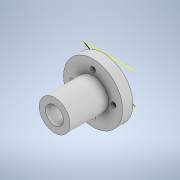
# Autodesk Inventor part: axis
Saved by Autodesk Inventor 2022 (Build 260153000, 153)
## iProperties
Created: 2023-10-26
Part Number: axis
Material: Generisch
Document SubType Name: Modeling
Designer: Marc Panse
Density: 1 g/cm^3
Appearance: Vorgabe
Author: Marc Panse
## iProperties of the stored document LCDmount_3D-Druck.ipt
Created: 2023-10-26
Part Number: LCDmount_3D-Druck
Material: Generisch
Document SubType Name: Modeling
Designer: Marc Panse
Density: 1 g/cm^3
Appearance: Vorgabe
Author: Marc Panse
Autodesk Inventor part; units mm, degrees
ref_plane "YZ Plane" through (0, 0, 0) normal (1, 0, 0) x (0, 1, 0)
ref_plane "XZ Plane" through (0, 0, 0) normal (0, 1, 0) x (-1, 0, 0)
ref_plane "XY Plane" through (0, 0, 0) normal (0, 0, 1) x (1, 0, 0)
sketch "Skizze1" plane through (0, 0, 0) normal (0, 0, 1) x (1, 0, 0)
  circle A0 centre (0, 0) radius 18
  circle A1 centre (0, 0) radius 25
  dimension "d0" = 36
  dimension "d1" = 50
  constraints: 2 centre point, 2 coincident
  measures "d0" diameter of A0
  measures "d1" diameter of A1
extrude "Extrusion1" add sketch "Skizze1" along normal blind 35
sketch "Skizze2" plane through (0, 0, 35) normal (0, 0, 1) x (1, 0, 0)
  circle A0 centre (0, 0) radius 19.3
  line L0 (0, -19.3) -> (0, -21.4)
  line L1 (0, -21.4) -> (-7.65, -21.4)
  line L2 (-7.65, -21.4) -> (7.65, -21.4)
  line L3 (7.65, -21.4) -> (7.65, -17.7191)
  line L4 (-7.65, -21.4) -> (-7.65, -17.7191)
  circle A1 centre (0, 0) radius 25 projected
  circle A2 centre (0, 0) radius 18 projected
  circle A3 centre (0, 0) radius 25 projected
  circle A4 centre (0, 0) radius 18 projected
  circle A5 centre (0, 0) radius 19.3
  dimension "d4" = 38.6
  dimension "d5" = 2.1
  dimension "d6" = 7.65
  dimension "d7" = 90
  dimension "d8" = 15.3
  constraints: 10 end point, 3 point on circle, 2 centre point, 2 coincident, 2 perpendicular, 1 concentric, 1 parallel, 1 point on line, 1 vertical
  measures "d4" diameter of A0
  measures "d5" distance of L0.start L0.end
  measures "d6" distance of L0.end L1.end
  measures "d7" angle of L0 L1
  measures "d8" distance of L1.end L2.end
extrude "Extrusion2" cut sketch "Skizze2" against normal blind 34 contours A0 | A0 L0 L1 L4 | L3 L2 L0 A0 | A2
fillet "Rundung1" radius 4 2 edges at (-7.65, -17.7191, 18) (7.65, -17.7191, 18)
sketch "Skizze3" plane through (0, 0, 35) normal (0, 0, 1) x (1, 0, 0)
  arc A0 (9.65, -16.7143) -> (7.65, -20.1784) centre (11.65, -20.1784) ccw projected
  line L0 (7.65, -20.1784) -> (7.65, -21.4) projected
  line L1 (7.65, -21.4) -> (-7.65, -21.4) projected
  line L2 (-7.65, -21.4) -> (-7.65, -20.1784) projected
  arc A1 (-7.65, -20.1784) -> (-9.65, -16.7143) centre (-11.65, -20.1784) ccw projected
  arc A2 (9.65, -16.7143) -> (-9.65, -16.7143) centre (0, 0) ccw projected
  circle A3 centre (0, 0) radius 25 projected
extrude "Extrusion3" cut sketch "Skizze3" against normal blind 25
sketch "Skizze4" plane through (0, 0, 10) normal (0, 0, 1) x (1, 0, 0)
  circle A0 centre (0, 0) radius 24
  circle A1 centre (0, 0) radius 25 projected
  arc A2 (9.65, -16.7143) -> (7.65, -20.1784) centre (11.65, -20.1784) ccw projected
  line L0 (7.65, -21.4) -> (7.65, -20.1784) projected
  line L1 (-7.65, -21.4) -> (7.65, -21.4) projected
  line L2 (-7.65, -20.1784) -> (-7.65, -21.4) projected
  arc A3 (-7.65, -20.1784) -> (-9.65, -16.7143) centre (-11.65, -20.1784) ccw projected
  arc A4 (9.65, -16.7143) -> (-9.65, -16.7143) centre (0, 0) ccw projected
  dimension "d14" = 48
  constraints: 1 centre point, 1 coincident
  measures "d14" diameter of A0
extrude "Extrusion4" cut sketch "Skizze4" against normal blind 9.25 contours A1
sketch "Skizze5" plane through (0, 0, 10) normal (0, 0, 1) x (1, 0, 0)
  circle A0 centre (0, 0) radius 24 projected
  arc A1 (9.65, -16.7143) -> (7.65, -20.1784) centre (11.65, -20.1784) ccw projected
  line L0 (7.65, -21.4) -> (7.65, -20.1784) projected
  line L1 (-7.65, -21.4) -> (7.65, -21.4) projected
  line L2 (-7.65, -20.1784) -> (-7.65, -21.4) projected
  arc A2 (-7.65, -20.1784) -> (-9.65, -16.7143) centre (-11.65, -20.1784) ccw projected
  arc A3 (9.65, -16.7143) -> (-9.65, -16.7143) centre (0, 0) ccw projected
extrude "Extrusion5" cut sketch "Skizze5" against normal blind 2.2
sketch "Skizze6" plane through (0, 0, 7.8) normal (0, 0, 1) x (1, 0, 0)
  line L0 (30, -2.706) -> (-30, -2.706)
  line L1 (-30, -2.706) -> (-30, 2.706)
  line L2 (-30, 2.706) -> (30, 2.706)
  line L3 (30, 2.706) -> (30, -2.706)
  line L4 (30, -2.706) -> (-30, 2.706) construction
  line L5 (-30, -2.706) -> (30, 2.706) construction
  point P0 (0, 0)
  dimension "d33" = 60
  constraints: 12 end point, 2 midpoint, 2 parallel, 1 horizontal, 1 perpendicular
  measures "d33" distance between parallel lines of L3 L1
extrude "Extrusion6" cut sketch "Skizze6" against normal blind 2.2
sketch "Skizze7" plane through (0, 0, 5.6) normal (0, 0, 1) x (1, 0, 0)
  line L0 (-22.5614, -2.035) -> (-22.5614, 2.035) projected
  line L1 (-22.5614, 0) -> (-19.3, 0)
  arc A0 (-19.1094, 2.706) -> (-19.1094, -2.706) centre (0, 0) ccw projected
  line L2 (-19.3, 0) -> (-24, 0)
  circle A1 centre (0, 0) radius 24 projected
  circle A2 centre (-21.65, 0) radius 0.9
  dimension "d34" = 1.8
  constraints: 4 end point, 2 horizontal, 2 midpoint, 1 centre point, 1 horizontal alignment, 1 point on circle, 1 other
  measures "d34" diameter of A2
extrude "Extrusion7" cut sketch "Skizze7" against normal blind 4 contours A2 L1 | L1 A2
mirror "Spiegeln1" about plane through (0, 0, 0) normal (1, 0, 0) of "Extrusion7"
sketch "Skizze8" plane through (0, 0, 7.8) normal (0, 0, 1) x (1, 0, 0)
  point P0 (0, 0)
pattern_circular "Runde Anordnung1" count 8 over 360 about axis through (0, 0, -10) along (0, 0, 1) of "Extrusion7", "Extrusion6"
sketch "Skizze9" plane through (0, -20.9307, 1.6) normal (0, 0, 1) x (1, 0, 0)
  line L0 (-0.8646, -0.4693) -> (0.8646, -0.4693) projected
  line L1 (-2.706, -0.4693) -> (-0.8646, -0.4693) projected
  line L2 (-2.706, 40.0401) -> (-2.706, 44.7777) projected
  line L3 (2.706, 44.7777) -> (2.706, 40.0401) projected
  arc A0 (2.706, 44.7777) -> (-2.706, 44.7777) centre (0, 20.9307) ccw projected
  arc A1 (2.706, 40.0401) -> (-2.706, 40.0401) centre (0, 20.9307) ccw projected
  arc A2 (-2.706, -2.9163) -> (2.706, -2.9163) centre (0, 20.9307) ccw projected
  line L4 (2.706, -0.4693) -> (2.706, -2.9163) projected
  line L5 (-2.706, -2.9163) -> (-2.706, -0.4693) projected
  line L6 (0.8646, -0.4693) -> (2.706, -0.4693) projected
  arc A3 (-0.8646, -0.4693) -> (0.8646, -0.4693) centre (0, -0.7193) ccw projected
  arc A4 (-0.8646, -0.4693) -> (0.8646, -0.4693) centre (0, -0.7193) ccw projected
extrude "Extrusion8" add sketch "Skizze9" along normal blind 4 contours L0 A3
sketch "Skizze10" plane through (-2.706, -21.4, 5.6) normal (0, 0, 1) x (1, 0, 0)
  line L0 (0, 0) -> (5.412, 0) projected
  line L1 (0, 40.5094) -> (0, 45.247) projected
  line L2 (5.412, 45.247) -> (5.412, 40.5094) projected
  arc A0 (5.412, 45.247) -> (0, 45.247) centre (2.706, 21.4) ccw projected
  arc A1 (5.412, 40.5094) -> (0, 40.5094) centre (2.706, 21.4) ccw projected
  arc A2 (0, -2.447) -> (5.412, -2.447) centre (2.706, 21.4) ccw projected
  line L3 (5.412, 0) -> (5.412, -2.447) projected
  line L4 (0, -2.447) -> (0, 0) projected
extrude "Extrusion9" add sketch "Skizze10" along normal up to surface (2.2 mm away)
sketch "Skizze11" plane through (0, 0, 7.8) normal (0, 0, 1) x (-0.3826834, -0.9238795, 0)
  line L0 (15.7149, 14.7896) -> (16.8435, 15.2571) projected
  arc A0 (11.7491, 15.3117) -> (9.8128, 16.6192) centre (0, 0) ccw projected
  line L1 (16.8435, 15.2571) -> (11.7491, 15.3117)
  line L2 (-18.6903, 4.8128) -> (-23.0673, 6.6258) projected
  arc A1 (9.8128, -16.6192) -> (16.6192, -9.8128) centre (0, 0) ccw projected
  line L3 (9.8128, -16.6192) -> (11.6258, -20.9962) projected
  line L4 (6.6258, -23.0673) -> (4.8128, -18.6903) projected
  arc A2 (-4.8128, -18.6903) -> (4.8128, -18.6903) centre (0, 0) ccw projected
  line L5 (-4.8128, -18.6903) -> (-6.6258, -23.0673) projected
  line L6 (4.8128, 18.6903) -> (6.6258, 23.0673) projected
  line L7 (20.9962, -11.6258) -> (16.6192, -9.8128) projected
  line L8 (18.6903, -4.8128) -> (23.0673, -6.6258) projected
  arc A3 (-9.8128, 16.6192) -> (-16.6192, 9.8128) centre (0, 0) ccw projected
  line L9 (-9.8128, 16.6192) -> (-11.6258, 20.9962) projected
  line L10 (-6.6258, 23.0673) -> (-4.8128, 18.6903) projected
  arc A4 (4.8128, 18.6903) -> (-4.8128, 18.6903) centre (0, 0) ccw projected
  line L11 (-11.6258, -20.9962) -> (-9.8128, -16.6192) projected
  line L12 (11.6258, 20.9962) -> (9.8128, 16.6192) projected
  arc A5 (11.7491, 15.3117) -> (9.8128, 16.6192) centre (0, 0) ccw projected
  arc A6 (11.7491, 15.3117) -> (15.7149, 14.7896) centre (14.1841, 18.4851) ccw projected
  line L13 (16.8435, 15.2571) -> (15.7149, 14.7896) projected
  line L14 (22.6986, 1.1217) -> (16.8435, 15.2571) projected
  line L15 (21.5699, 0.6543) -> (22.6986, 1.1217) projected
  arc A7 (21.5699, 0.6543) -> (19.1349, -2.5192) centre (23.1007, -3.0413) ccw projected
  arc A8 (18.6903, -4.8128) -> (19.1349, -2.5192) centre (0, 0) ccw projected
  line L16 (-20.9962, 11.6258) -> (-16.6192, 9.8128) projected
  arc A9 (-6.6258, -23.0673) -> (6.6258, -23.0673) centre (0, 0) ccw projected
  arc A10 (-18.6903, 4.8128) -> (-9.8128, -16.6192) centre (0, 0) ccw projected
  arc A11 (-23.0673, 6.6258) -> (-11.6258, -20.9962) centre (0, 0) ccw projected
  arc A12 (-11.6258, 20.9962) -> (-20.9962, 11.6258) centre (0, 0) ccw projected
  arc A13 (11.6258, -20.9962) -> (20.9962, -11.6258) centre (0, 0) ccw projected
  arc A14 (6.6258, 23.0673) -> (-6.6258, 23.0673) centre (0, 0) ccw projected
  arc A15 (23.0673, -6.6258) -> (11.6258, 20.9962) centre (0, 0) ccw projected
  point P0 (15.7149, 14.7896)
  constraints: 2 end point
extrude "Extrusion10" cut sketch "Skizze11" against normal up to surface (6.8 mm away) contours A6 L1 L0
mirror "Spiegeln2" about plane through (0, 0, 0) normal (1, 0, 0) of "Extrusion10"
sketch "Skizze12" plane through (0, 0, 7.8) normal (0, 0, 1) x (-0.3826834, -0.9238795, 0)
  point P0 (0, 0)
sketch "Skizze13" plane through (0, 0, 7.8) normal (0, 0, 1) x (1, 0, 0)
  line L0 (-7.65, -21.4) -> (-9.65, -16.7143) projected
  arc A0 (-11.5989, -15.4258) -> (-9.65, -16.7143) centre (0, 0) ccw projected
  line L1 (-11.5989, -15.4258) -> (-14.9489, -18.7758) projected
  arc A1 (-14.9489, -18.7758) -> (14.9489, -18.7758) centre (0, 0) ccw projected
  line L2 (14.9489, -18.7758) -> (11.5989, -15.4258) projected
  arc A2 (9.65, -16.7143) -> (11.5989, -15.4258) centre (0, 0) ccw projected
  line L3 (9.65, -16.7143) -> (7.65, -21.4) projected
  line L4 (-7.65, -21.4) -> (7.65, -21.4) projected
  arc A3 (-11.5989, -15.4258) -> (-9.65, -16.7143) centre (0, 0) ccw projected
  line L5 (7.65, -21.4) -> (-7.65, -21.4) projected
  line L6 (-11.5989, -15.4258) -> (-7.65, -21.4)
  constraints: 2 end point
extrude "Extrusion11" cut sketch "Skizze13" against normal up to surface (6.8 mm away) contours L6 A0 L0
mirror "Spiegeln3" about plane through (0, 0, 0) normal (1, 0, 0) of "Extrusion11"
sketch "Skizze14" plane through (0, 0, 1) normal (0, 0, 1) x (1, 0, 0)
  point P0 (0, 0)
sketch "Skizze15" plane through (0, 0, 7.8) normal (0, 0, 1) x (1, 0, 0)
  circle A0 centre (0, 0) radius 19.375
  dimension "d37" = 38.75
  constraints: 1 centre point, 1 coincident
  measures "d37" diameter of A0
extrude "Extrusion12" cut sketch "Skizze15" against normal up to surface (7.05 mm away)
sketch "Skizze16" plane through (0, 0, 7.8) normal (0, 0, 1) x (1, 0, 0)
  line L0 (29.93, -29.5015) -> (-37.5684, -24.9946) construction
  line L1 (-37.5684, -24.9946) -> (-33.6707, 33.3801) construction
  line L2 (-33.6707, 33.3801) -> (33.8277, 28.8732) construction
  line L3 (33.8277, 28.8732) -> (29.93, -29.5015) construction
  point P0 (0, 0)
  constraints: 2 other
sketch "Skizze18" plane through (0, 0, 5.6) normal (0, 0, 1) x (0.7071068, -0.7071068, 0)
  circle A0 centre (-21.65, 0) radius 0.9 projected
  arc A1 (-19.1851, 2.706) -> (-19.1851, -2.706) centre (0, 0) ccw projected
  line L0 (-23.847, 2.706) -> (-19.1851, 2.706) projected
  arc A2 (-23.847, 2.706) -> (-23.847, -2.706) centre (0, 0) ccw projected
  line L1 (-19.1851, -2.706) -> (-23.847, -2.706) projected
  arc A3 (19.1851, -2.706) -> (19.1851, 2.706) centre (0, 0) ccw projected
  line L2 (23.847, -2.706) -> (19.1851, -2.706) projected
  arc A4 (23.847, -2.706) -> (23.847, 2.706) centre (0, 0) ccw projected
  line L3 (19.1851, 2.706) -> (23.847, 2.706) projected
  circle A5 centre (21.65, 0) radius 0.9 projected
  arc A6 (15.4793, 11.6525) -> (11.6525, 15.4793) centre (0, 0) ccw projected
  line L4 (18.7758, 14.9489) -> (15.4793, 11.6525) projected
  arc A7 (18.7758, 14.9489) -> (14.9489, 18.7758) centre (0, 0) ccw projected
  line L5 (11.6525, 15.4793) -> (14.9489, 18.7758) projected
  circle A8 centre (15.3089, 15.3089) radius 0.9 projected
  circle A9 centre (0, 21.65) radius 0.9 projected
  arc A10 (2.706, 19.1851) -> (-2.706, 19.1851) centre (0, 0) ccw projected
  line L6 (2.706, 23.847) -> (2.706, 19.1851) projected
  arc A11 (2.706, 23.847) -> (-2.706, 23.847) centre (0, 0) ccw projected
  line L7 (-2.706, 19.1851) -> (-2.706, 23.847) projected
  arc A12 (-2.706, -19.1851) -> (2.706, -19.1851) centre (0, 0) ccw projected
  line L8 (-2.706, -23.847) -> (-2.706, -19.1851) projected
  arc A13 (-2.706, -23.847) -> (2.706, -23.847) centre (0, 0) ccw projected
  line L9 (2.706, -19.1851) -> (2.706, -23.847) projected
  circle A14 centre (0, -21.65) radius 0.9 projected
  arc A15 (-15.4793, -11.6525) -> (-11.6525, -15.4793) centre (0, 0) ccw projected
  line L10 (-18.7758, -14.9489) -> (-15.4793, -11.6525) projected
  arc A16 (-18.7758, -14.9489) -> (-14.9489, -18.7758) centre (0, 0) ccw projected
  line L11 (-11.6525, -15.4793) -> (-14.9489, -18.7758) projected
  circle A17 centre (-15.3089, -15.3089) radius 0.9 projected
  line L12 (23.847, -2.706) -> (19.1851, -2.706) projected
  line L13 (-23.847, -2.706) -> (23.847, -2.706)
  line L14 (19.1851, 2.706) -> (23.847, 2.706) projected
  line L15 (-23.847, 2.706) -> (23.847, 2.706)
  line L16 (-2.706, 23.847) -> (-2.706, -23.847)
  arc A18 (-2.706, -23.847) -> (2.706, -23.847) centre (0, 0) ccw projected
  line L17 (2.706, 23.847) -> (2.706, -23.847)
  line L18 (11.6525, 15.4793) -> (14.9489, 18.7758) projected
  line L19 (-18.7758, -14.9489) -> (14.9489, 18.7758)
  line L20 (-14.9489, -18.7758) -> (18.7758, 14.9489)
  point P0 (-19.1851, -2.706)
  point P1 (19.1851, -2.706)
  point P2 (19.1851, 2.706)
  point P3 (-19.1851, 2.706)
  point P4 (6.5328, 2.706)
  point P5 (15.4793, 11.6525)
  point P6 (11.6525, 15.4793)
  point P7 (2.706, 6.5328)
  point P8 (-2.706, 19.1851)
  point P9 (-2.706, 2.706)
  point P10 (-2.706, -6.5328)
  point P11 (2.706, -19.1851)
  point P12 (2.706, -2.706)
  point P13 (-6.5328, -2.706)
  point P14 (-15.4793, -11.6525)
  point P15 (-11.6525, -15.4793)
  constraints: 12 end point, 2 horizontal, 2 vertical, 1 collinear
extrude "Extrusion13" add sketch "Skizze18" along normal blind 4
sketch "Skizze19" plane through (0, 0, 9.6) normal (0, 0, 1) x (0.7071068, 0.7071068, 0)
  circle A0 centre (0, 0) radius 19.375
  constraints: 1 centre point, 1 coincident
extrude "Extrusion14" add sketch "Skizze19" against normal blind 4
sketch "Skizze20" plane through (0, 0, 9.6) normal (0, 0, 1) x (0.7071068, 0.7071068, 0)
  line L0 (-2.7577, 15.8392) -> (15.8392, -2.7577)
  line L1 (15.8392, -2.7577) -> (2.7577, -15.8392)
  line L2 (2.7577, -15.8392) -> (-15.8392, 2.7577)
  line L3 (-15.8392, 2.7577) -> (-2.7577, 15.8392)
  line L4 (-2.7577, 15.8392) -> (2.7577, -15.8392) construction
  line L5 (15.8392, -2.7577) -> (-15.8392, 2.7577) construction
  line L6 (-2.7577, 15.8392) -> (23.5423, 15.8392) construction
  circle A0 centre (-2.7577, 15.8392) radius 1
  circle A1 centre (15.8392, -2.7577) radius 1
  circle A2 centre (2.7577, -15.8392) radius 1
  circle A3 centre (-15.8392, 2.7577) radius 1
  line L7 (6.5407, 6.5407) -> (13.6118, -0.5303)
  line L8 (13.6118, -0.5303) -> (-0.5303, 13.6118)
  line L9 (-0.5303, 13.6118) -> (-9.0156, 5.1265)
  line L10 (-9.0156, 5.1265) -> (5.1265, -9.0156)
  line L11 (5.1265, -9.0156) -> (13.6118, -0.5303)
  point P0 (0, 0)
  dimension "d68" = 45
  dimension "d69" = 18.5
  dimension "d70" = 26.3
  dimension "d71" = 2
  dimension "d72" = 2
  dimension "d73" = 2
  dimension "d74" = 2
  dimension "d75" = 10
  dimension "d76" = 20
  dimension "d77" = 12
  constraints: 24 end point, 4 centre point, 4 perpendicular, 3 coincident, 3 midpoint, 3 point on line, 2 parallel, 1 equal length, 1 horizontal
  measures "d68" angle of L0 L6
  measures "d69" distance of L0.end L1.end
  measures "d70" distance between parallel lines of L1 L3
  measures "d71" diameter of A0
  measures "d72" diameter of A1
  measures "d73" diameter of A2
  measures "d74" diameter of A3
  measures "d75" distance of L7.start L7.end
  measures "d76" distance of L7.end L8.end
  measures "d77" distance of L8.end L9.end
extrude "Extrusion15" cut sketch "Skizze20" against normal blind 10 contours L0 L11 L10 L9 | A0 L3 L0 | L0 L3 A0 | A1 L1 L0 | L0 L1 A1 | A3 L2 L3 | L3 L2 A3 | A2 L2 L1 | L1 L2 A2
sketch "Skizze21" plane through (0, 0, 0) normal (0, 0, -1) x (-1, 0, 0)
  circle A0 centre (0, 0) radius 36.2335
  constraints: 1 centre point, 1 coincident
extrude "Extrusion16" cut sketch "Skizze21" against normal up to surface (7.8 mm away)
sketch "Skizze22" plane through (0, 0, 9.6) normal (0, 0, 1) x (0.7071068, 0.7071068, 0)
  line L0 (-0.5303, 13.6118) -> (13.6118, -0.5303) projected
  line L1 (-0.5303, 13.6118) -> (5.1265, -9.0156)
  point P0 (0, 0)
  constraints: 2 end point
sketch "Skizze23" plane through (0, 0, 9.6) normal (0, 0, 1) x (0.7071068, 0.7071068, 0)
  line L0 (-0.5303, 13.6118) -> (5.1265, -9.0156) projected
  line L1 (-0.5303, 13.6118) -> (13.6118, -0.5303)
  line L2 (13.6118, -0.5303) -> (5.1265, -9.0156)
  line L3 (5.1265, -9.0156) -> (-9.0156, 5.1265)
  line L4 (-9.0156, 5.1265) -> (-0.5303, 13.6118)
  line L5 (-0.5303, 13.6118) -> (5.1265, -9.0156) construction
  line L6 (13.6118, -0.5303) -> (-9.0156, 5.1265) construction
  point P0 (0, 0)
  point P1 (2.2981, 2.2981)
  constraints: 12 end point, 3 midpoint, 2 parallel, 1 perpendicular
extrude "Extrusion17" add sketch "Skizze23" against normal blind 0.5
sketch "Skizze24" plane through (0, 0, 9.6) normal (0, 0, 1) x (0.7071068, 0.7071068, 0)
  circle A0 centre (15.8392, -2.7577) radius 1 projected
  circle A1 centre (2.7577, -15.8392) radius 1 projected
  circle A2 centre (-15.8392, 2.7577) radius 1 projected
  circle A3 centre (-2.7577, 15.8392) radius 1 projected
  circle A4 centre (0, 21.65) radius 0.9 projected
  circle A5 centre (-15.3089, 15.3089) radius 0.9 projected
  circle A6 centre (-21.65, 0) radius 0.9 projected
  circle A7 centre (0, -21.65) radius 0.9 projected
  circle A8 centre (15.3089, -15.3089) radius 0.9 projected
  circle A9 centre (21.65, 0) radius 0.9 projected
  arc A10 (19.1851, 2.706) -> (2.706, 19.1851) centre (0, 0) ccw projected
  line L0 (2.706, 19.1851) -> (2.706, 23.847) projected
  arc A11 (2.706, 23.847) -> (-2.706, 23.847) centre (0, 0) ccw projected
  line L1 (-2.706, 23.847) -> (-2.706, 19.1851) projected
  arc A12 (-2.706, 19.1851) -> (-11.6525, 15.4793) centre (0, 0) ccw projected
  line L2 (-11.6525, 15.4793) -> (-14.9489, 18.7758) projected
  arc A13 (-14.9489, 18.7758) -> (-18.7758, 14.9489) centre (0, 0) ccw projected
  line L3 (-18.7758, 14.9489) -> (-15.4793, 11.6525) projected
  arc A14 (-15.4793, 11.6525) -> (-19.1851, 2.706) centre (0, 0) ccw projected
  line L4 (-19.1851, 2.706) -> (-23.847, 2.706) projected
  arc A15 (-23.847, 2.706) -> (-23.847, -2.706) centre (0, 0) ccw projected
  line L5 (-23.847, -2.706) -> (-19.1851, -2.706) projected
  arc A16 (-19.1851, -2.706) -> (-2.706, -19.1851) centre (0, 0) ccw projected
  line L6 (-2.706, -19.1851) -> (-2.706, -23.847) projected
  arc A17 (-2.706, -23.847) -> (2.706, -23.847) centre (0, 0) ccw projected
  line L7 (2.706, -23.847) -> (2.706, -19.1851) projected
  arc A18 (2.706, -19.1851) -> (11.6525, -15.4793) centre (0, 0) ccw projected
  line L8 (11.6525, -15.4793) -> (14.9489, -18.7758) projected
  arc A19 (14.9489, -18.7758) -> (18.7758, -14.9489) centre (0, 0) ccw projected
  line L9 (18.7758, -14.9489) -> (15.4793, -11.6525) projected
  arc A20 (15.4793, -11.6525) -> (19.1851, -2.706) centre (0, 0) ccw projected
  line L10 (19.1851, -2.706) -> (23.847, -2.706) projected
  arc A21 (23.847, -2.706) -> (23.847, 2.706) centre (0, 0) ccw projected
  line L11 (23.847, 2.706) -> (19.1851, 2.706) projected
extrude "Extrusion18" add sketch "Skizze24" along normal blind 2.3
sketch "Skizze25" plane through (0, 0, 7.8) normal (0, 0, -1) x (-1, 0, 0)
  circle A0 centre (0, 0) radius 5
  dimension "d86" = 10
  constraints: 1 centre point, 1 coincident
  measures "d86" diameter of A0
extrude "Extrusion19" cut sketch "Skizze25" against normal blind 30
sketch "Skizze26" plane through (0, 0, 7.8) normal (0, 0, -1) x (-1, 0, 0)
  arc A0 (-4.1758, -2.75) -> (4.1758, -2.75) centre (0, 0) ccw projected
  line L0 (-10, -2.75) -> (-4.1758, -2.75) projected
  line L1 (-10, 9.25) -> (-10, -2.75) projected
  line L2 (10, 9.25) -> (-10, 9.25) projected
  line L3 (10, -2.75) -> (10, 9.25) projected
  line L4 (4.1758, -2.75) -> (10, -2.75) projected
  circle A1 centre (-13.15, 9.25) radius 1 projected
  circle A2 centre (-13.15, -9.25) radius 1 projected
  circle A3 centre (13.15, -9.25) radius 1 projected
  circle A4 centre (13.15, 9.25) radius 1 projected
  arc A5 (11.6525, 15.4793) -> (-11.6525, 15.4793) centre (0, 0) ccw projected
  line L5 (-11.6525, 15.4793) -> (-14.9489, 18.7758) projected
  arc A6 (-14.9489, 18.7758) -> (-18.7758, 14.9489) centre (0, 0) ccw projected
  line L6 (-18.7758, 14.9489) -> (-15.4793, 11.6525) projected
  arc A7 (-15.4793, 11.6525) -> (-19.1851, 2.706) centre (0, 0) ccw projected
  line L7 (-19.1851, 2.706) -> (-23.847, 2.706) projected
  arc A8 (-23.847, 2.706) -> (-23.847, -2.706) centre (0, 0) ccw projected
  line L8 (-23.847, -2.706) -> (-19.1851, -2.706) projected
  arc A9 (-19.1851, -2.706) -> (-15.4793, -11.6525) centre (0, 0) ccw projected
  line L9 (-15.4793, -11.6525) -> (-18.7758, -14.9489) projected
  arc A10 (-18.7758, -14.9489) -> (-14.9489, -18.7758) centre (0, 0) ccw projected
  line L10 (-14.9489, -18.7758) -> (-11.6525, -15.4793) projected
  arc A11 (-11.6525, -15.4793) -> (11.6525, -15.4793) centre (0, 0) ccw projected
  line L11 (11.6525, -15.4793) -> (14.9489, -18.7758) projected
  arc A12 (14.9489, -18.7758) -> (18.7758, -14.9489) centre (0, 0) ccw projected
  line L12 (18.7758, -14.9489) -> (15.4793, -11.6525) projected
  arc A13 (15.4793, -11.6525) -> (19.1851, -2.706) centre (0, 0) ccw projected
  line L13 (19.1851, -2.706) -> (23.847, -2.706) projected
  arc A14 (23.847, -2.706) -> (23.847, 2.706) centre (0, 0) ccw projected
  line L14 (23.847, 2.706) -> (19.1851, 2.706) projected
  arc A15 (19.1851, 2.706) -> (15.4793, 11.6525) centre (0, 0) ccw projected
  line L15 (15.4793, 11.6525) -> (18.7758, 14.9489) projected
  arc A16 (18.7758, 14.9489) -> (14.9489, 18.7758) centre (0, 0) ccw projected
  line L16 (14.9489, 18.7758) -> (11.6525, 15.4793) projected
  circle A17 centre (21.65, 0) radius 0.9 projected
  circle A18 centre (-21.65, 0) radius 0.9 projected
  circle A19 centre (15.3089, -15.3089) radius 0.9 projected
  circle A20 centre (-15.3089, -15.3089) radius 0.9 projected
  circle A21 centre (-15.3089, 15.3089) radius 0.9 projected
  circle A22 centre (15.3089, 15.3089) radius 0.9 projected
  circle A23 centre (0, 0) radius 19.375
  point P0 (15.4793, -11.6525)
  point P1 (11.6525, -15.4793)
  point P2 (19.1851, 2.706)
  point P3 (19.1851, -2.706)
  point P4 (11.6525, 15.4793)
  point P5 (15.4793, 11.6525)
  point P6 (-11.6525, -15.4793)
  point P7 (-15.4793, -11.6525)
  point P8 (-19.1851, -2.706)
  point P9 (-19.1851, 2.706)
  point P10 (-15.4793, 11.6525)
  point P11 (-11.6525, 15.4793)
  constraints: 1 centre point, 1 coincident
extrude "Extrusion20" add sketch "Skizze26" along normal blind 4 contours L16 A16 L15 A23 | A23 L6 A6 L5 | L14 A14 L13 A23 | A23 L8 A8 L7 | A23 L10 A10 L9 | L12 A12 L11 A23
sketch "Skizze27" plane through (0, 0, 7.8) normal (0, 0, -1) x (-1, 0, 0)
  line L0 (0, 0) -> (0, 8)
  line L1 (0, 8) -> (0, -8)
  line L2 (0, 0) -> (8, 0)
  line L3 (8, 0) -> (-8, 0)
  circle A0 centre (-8, 0) radius 1
  circle A1 centre (0, 8) radius 1
  circle A2 centre (0, -8) radius 1
  circle A3 centre (8, 0) radius 1
  dimension "d91" = 8
  dimension "d92" = 16
  dimension "d93" = 8
  dimension "d94" = 16
  dimension "d95" = 2
  dimension "d96" = 2
  dimension "d97" = 2
  dimension "d98" = 2
  constraints: 8 end point, 4 centre point, 4 coincident, 2 point on line, 1 horizontal, 1 vertical
  measures "d91" distance of L0.start L0.end
  measures "d92" distance of L0.end L1.end
  measures "d93" distance of L0.start L2.end
  measures "d94" distance of L2.end L3.end
  measures "d95" diameter of A0
  measures "d96" diameter of A1
  measures "d97" diameter of A2
  measures "d98" diameter of A3
extrude "Extrusion21" cut sketch "Skizze27" against normal blind 29.5
sketch "Skizze28" plane through (0, 0, 7.8) normal (0, 0, -1) x (-1, 0, 0)
  point P0 (0, 0)
sketch "Skizze29" plane through (0, 0, 7.8) normal (0, 0, -1) x (-1, 0, 0)
  line L0 (11.6525, 15.4793) -> (14.9489, 18.7758)
  circle A0 centre (0, 0) radius 24
  circle A1 centre (0, -8) radius 1
  arc A2 (-15.4793, -11.6525) -> (-11.6525, -15.4793) centre (0, 0) ccw
  arc A3 (-11.6525, -15.4793) -> (11.6525, -15.4793) centre (0, 0) ccw
  arc A4 (11.6525, -15.4793) -> (15.4793, -11.6525) centre (0, 0) ccw
  arc A5 (15.4793, -11.6525) -> (19.1851, -2.706) centre (0, 0) ccw
  arc A6 (19.1851, -2.706) -> (19.1851, 2.706) centre (0, 0) ccw
  arc A7 (19.1851, 2.706) -> (15.4793, 11.6525) centre (0, 0) ccw
  arc A8 (15.4793, 11.6525) -> (11.6525, 15.4793) centre (0, 0) ccw
  arc A9 (11.6525, 15.4793) -> (-11.6525, 15.4793) centre (0, 0) ccw
  arc A10 (-11.6525, 15.4793) -> (-15.4793, 11.6525) centre (0, 0) ccw
  arc A11 (-15.4793, 11.6525) -> (-19.1851, 2.706) centre (0, 0) ccw
  arc A12 (-19.1851, 2.706) -> (-19.1851, -2.706) centre (0, 0) ccw
  arc A13 (-19.1851, -2.706) -> (-15.4793, -11.6525) centre (0, 0) ccw
  circle A14 centre (13.15, 9.25) radius 1
  circle A15 centre (13.15, -9.25) radius 1
  circle A16 centre (-13.15, -9.25) radius 1
  circle A17 centre (-13.15, 9.25) radius 1
  arc A18 (-4.1758, -2.75) -> (4.1758, -2.75) centre (0, 0) ccw
  line L1 (-10, -2.75) -> (-4.1758, -2.75)
  line L2 (-10, 9.25) -> (-10, -2.75)
  line L3 (10, 9.25) -> (-10, 9.25)
  line L4 (10, -2.75) -> (10, 9.25)
  line L5 (4.1758, -2.75) -> (10, -2.75)
  line L6 (-18.7758, 14.9489) -> (-15.4793, 11.6525)
  arc A19 (-11.6525, 15.4793) -> (-15.4793, 11.6525) centre (0, 0) ccw
  line L7 (-11.6525, 15.4793) -> (-14.9489, 18.7758)
  arc A20 (-14.9489, 18.7758) -> (-18.7758, 14.9489) centre (0, 0) ccw
  circle A21 centre (-15.3089, 15.3089) radius 0.9
  line L8 (14.9489, 18.7758) -> (11.6525, 15.4793)
  arc A22 (15.4793, 11.6525) -> (11.6525, 15.4793) centre (0, 0) ccw
  line L9 (15.4793, 11.6525) -> (18.7758, 14.9489)
  arc A23 (18.7758, 14.9489) -> (14.9489, 18.7758) centre (0, 0) ccw
  circle A24 centre (15.3089, 15.3089) radius 0.9
  line L10 (-14.9489, -18.7758) -> (-11.6525, -15.4793)
  arc A25 (-15.4793, -11.6525) -> (-11.6525, -15.4793) centre (0, 0) ccw
  line L11 (-15.4793, -11.6525) -> (-18.7758, -14.9489)
  arc A26 (-18.7758, -14.9489) -> (-14.9489, -18.7758) centre (0, 0) ccw
  circle A27 centre (-15.3089, -15.3089) radius 0.9
  line L12 (-23.847, -2.706) -> (-19.1851, -2.706)
  arc A28 (-19.1851, 2.706) -> (-19.1851, -2.706) centre (0, 0) ccw
  line L13 (-19.1851, 2.706) -> (-23.847, 2.706)
  arc A29 (-23.847, 2.706) -> (-23.847, -2.706) centre (0, 0) ccw
  circle A30 centre (-21.65, 0) radius 0.9
  line L14 (23.847, 2.706) -> (19.1851, 2.706)
  arc A31 (19.1851, -2.706) -> (19.1851, 2.706) centre (0, 0) ccw
  line L15 (19.1851, -2.706) -> (23.847, -2.706)
  arc A32 (23.847, -2.706) -> (23.847, 2.706) centre (0, 0) ccw
  circle A33 centre (21.65, 0) radius 0.9
  line L16 (18.7758, -14.9489) -> (15.4793, -11.6525)
  arc A34 (11.6525, -15.4793) -> (15.4793, -11.6525) centre (0, 0) ccw
  line L17 (11.6525, -15.4793) -> (14.9489, -18.7758)
  arc A35 (14.9489, -18.7758) -> (18.7758, -14.9489) centre (0, 0) ccw
  circle A36 centre (15.3089, -15.3089) radius 0.9
  point P0 (15.4793, 11.6525)
  point P1 (19.1851, 2.706)
  point P2 (18.7758, 14.9489)
  point P3 (19.1851, -2.706)
  point P4 (15.4793, -11.6525)
  point P5 (23.847, -2.706)
  point P6 (11.6525, -15.4793)
  point P7 (-11.6525, -15.4793)
  point P8 (14.9489, -18.7758)
  point P9 (-15.4793, -11.6525)
  point P10 (-19.1851, -2.706)
  point P11 (-18.7758, -14.9489)
  point P12 (-19.1851, 2.706)
  point P13 (-15.4793, 11.6525)
  point P14 (-23.847, 2.706)
  point P15 (-11.6525, 15.4793)
  point P16 (-14.9489, 18.7758)
extrude "Extrusion22" add sketch "Skizze29" along normal blind 1.7 contours A9 L7 A0 L0 | L9 A0 L14 A7 | A11 L13 A0 L6 | L15 A0 L16 A5 | A13 L11 A0 L12 | L17 A0 L10 A3
sketch "Skizze30" plane through (0, 0, 7.8) normal (0, 0, -1) x (-1, 0, 0)
  circle A0 centre (13.15, 9.25) radius 1 projected
  circle A1 centre (13.15, 9.25) radius 1.5
  circle A2 centre (13.15, -9.25) radius 1 projected
  circle A3 centre (13.15, -9.25) radius 1.5
  circle A4 centre (-13.15, -9.25) radius 1 projected
  circle A5 centre (-13.15, -9.25) radius 1.5
  circle A6 centre (-13.15, 9.25) radius 1 projected
  circle A7 centre (-13.15, 9.25) radius 1.5
  point P0 (0, 0)
  dimension "d103" = 3
  dimension "d104" = 3
  dimension "d105" = 3
  dimension "d106" = 3
  constraints: 4 centre point, 4 coincident
  measures "d103" diameter of A1
  measures "d104" diameter of A3
  measures "d105" diameter of A5
  measures "d106" diameter of A7
extrude "Extrusion23" add sketch "Skizze30" along normal blind 1.7
sketch "Skizze31" plane through (0, 0, 11.9) normal (0, 0, 1) x (0.7071068, -0.7071068, 0)
  point P0 (0, 0)
sketch "Skizze32" plane through (0, 0, 7.8) normal (0, 0, 1) x (1, 0, 0)
  line L0 (14.9489, 18.7758) -> (11.6525, 15.4793) projected
  circle A0 centre (0, 0) radius 19.375
  arc A1 (14.9489, 18.7758) -> (-14.9489, 18.7758) centre (0, 0) ccw projected
  circle A2 centre (0, 0) radius 24
  circle A3 centre (-8, 0) radius 1 projected
  circle A4 centre (0, 8) radius 1 projected
  circle A5 centre (0, -8) radius 1 projected
  circle A6 centre (8, 0) radius 1 projected
  circle A7 centre (0, 0) radius 5 projected
  line L1 (-11.6525, 15.4793) -> (-14.9489, 18.7758) projected
  arc A8 (-14.9489, 18.7758) -> (-18.7758, 14.9489) centre (0, 0) ccw projected
  line L2 (-18.7758, 14.9489) -> (-15.4793, 11.6525) projected
  arc A9 (-15.4793, 11.6525) -> (-19.1851, 2.706) centre (0, 0) ccw projected
  line L3 (-19.1851, 2.706) -> (-23.847, 2.706) projected
  arc A10 (-23.847, 2.706) -> (-23.847, -2.706) centre (0, 0) ccw projected
  line L4 (-23.847, -2.706) -> (-19.1851, -2.706) projected
  arc A11 (-19.1851, -2.706) -> (-15.4793, -11.6525) centre (0, 0) ccw projected
  line L5 (-15.4793, -11.6525) -> (-18.7758, -14.9489) projected
  arc A12 (-18.7758, -14.9489) -> (-14.9489, -18.7758) centre (0, 0) ccw projected
  line L6 (-14.9489, -18.7758) -> (-11.6525, -15.4793) projected
  arc A13 (-11.6525, -15.4793) -> (11.6525, -15.4793) centre (0, 0) ccw projected
  line L7 (11.6525, -15.4793) -> (14.9489, -18.7758) projected
  arc A14 (14.9489, -18.7758) -> (18.7758, -14.9489) centre (0, 0) ccw projected
  line L8 (18.7758, -14.9489) -> (15.4793, -11.6525) projected
  arc A15 (15.4793, -11.6525) -> (19.1851, -2.706) centre (0, 0) ccw projected
  line L9 (19.1851, -2.706) -> (23.847, -2.706) projected
  arc A16 (23.847, -2.706) -> (23.847, 2.706) centre (0, 0) ccw projected
  line L10 (23.847, 2.706) -> (19.1851, 2.706) projected
  arc A17 (19.1851, 2.706) -> (15.4793, 11.6525) centre (0, 0) ccw projected
  line L11 (15.4793, 11.6525) -> (18.7758, 14.9489) projected
  arc A18 (18.7758, 14.9489) -> (14.9489, 18.7758) centre (0, 0) ccw projected
  line L12 (14.9489, 18.7758) -> (11.6525, 15.4793) projected
  arc A19 (11.6525, 15.4793) -> (-11.6525, 15.4793) centre (0, 0) ccw projected
  circle A20 centre (13.15, 9.25) radius 1 projected
  circle A21 centre (13.15, -9.25) radius 1 projected
  circle A22 centre (-13.15, -9.25) radius 1 projected
  circle A23 centre (-13.15, 9.25) radius 1 projected
  circle A24 centre (-21.65, 0) radius 0.9 projected
  circle A25 centre (21.65, 0) radius 0.9 projected
  circle A26 centre (15.3089, 15.3089) radius 0.9 projected
  circle A27 centre (15.3089, -15.3089) radius 0.9 projected
  circle A28 centre (-15.3089, -15.3089) radius 0.9 projected
  circle A29 centre (-15.3089, 15.3089) radius 0.9 projected
  point P0 (18.7758, 14.9489)
  point P1 (15.4793, 11.6525)
  point P2 (19.1851, 2.706)
  point P3 (23.847, 2.706)
  point P4 (23.847, -2.706)
  point P5 (19.1851, -2.706)
  point P6 (15.4793, -11.6525)
  point P7 (18.7758, -14.9489)
  point P8 (14.9489, -18.7758)
  point P9 (11.6525, -15.4793)
  point P10 (-11.6525, -15.4793)
  point P11 (-14.9489, -18.7758)
  point P12 (-18.7758, -14.9489)
  point P13 (-15.4793, -11.6525)
  point P14 (-19.1851, -2.706)
  point P15 (-23.847, -2.706)
  point P16 (-23.847, 2.706)
  point P17 (-19.1851, 2.706)
  point P18 (-15.4793, 11.6525)
  point P19 (-18.7758, 14.9489)
  point P20 (-14.9489, 18.7758)
  constraints: 2 coincident, 6 other
extrude "Extrusion24" add sketch "Skizze32" along normal up to surface (4.1 mm away) contours L0 A0 L1 A1 | A2 L10 A0 L11 | L2 A0 L3 A2 | L4 A0 L5 A2 | A2 L8 A0 L9 | L6 A0 L7 A2
sketch "Skizze33" plane through (-13.15, 9.25, 6.1) normal (0, 0, -1) x (-1, 0, 0)
  circle A0 centre (-26.3, 0) radius 1 projected
  circle A1 centre (0, 0) radius 1 projected
  circle A2 centre (0, -18.5) radius 1 projected
  circle A3 centre (-26.3, -18.5) radius 1 projected
  point P0 (-13.15, -9.25)
extrude "Extrusion25" add sketch "Skizze33" against normal up to surface (5.8 mm away)
sketch "Skizze34" plane through (0, 0, 11.9) normal (0, 0, 1) x (1, 0, 0)
  circle A0 centre (0, 0) radius 11.5
  circle A1 centre (-8, 0) radius 1 projected
  circle A2 centre (0, 8) radius 1 projected
  circle A3 centre (0, -8) radius 1 projected
  circle A4 centre (8, 0) radius 1 projected
  circle A5 centre (0, 0) radius 5 projected
  circle A6 centre (0, 0) radius 24 projected
  circle A7 centre (-21.65, 0) radius 0.9 projected
  circle A8 centre (21.65, 0) radius 0.9 projected
  circle A9 centre (15.3089, 15.3089) radius 0.9 projected
  circle A10 centre (15.3089, -15.3089) radius 0.9 projected
  circle A11 centre (-15.3089, -15.3089) radius 0.9 projected
  circle A12 centre (-15.3089, 15.3089) radius 0.9 projected
  dimension "d113" = 23
  constraints: 1 centre point, 1 coincident
  measures "d113" diameter of A0
extrude "Extrusion26" add sketch "Skizze34" along normal blind 4 contours A0
sketch "Skizze35" plane through (0, 0, 15.9) normal (0, 0, 1) x (1, 0, 0)
  circle A0 centre (0, 0) radius 6
  circle A1 centre (0, 0) radius 11.5 projected
  circle A2 centre (0, 0) radius 5 projected
  circle A3 centre (8, 0) radius 1 projected
  circle A4 centre (0, -8) radius 1 projected
  circle A5 centre (0, 8) radius 1 projected
  circle A6 centre (-8, 0) radius 1 projected
  dimension "d116" = 12
  constraints: 1 centre point, 1 coincident
  measures "d116" diameter of A0
extrude "Extrusion27" add sketch "Skizze35" along normal blind 15 contours A0
sketch "Skizze36" plane through (0, 0, 30.9) normal (0, 0, 1) x (1, 0, 0)
  circle A0 centre (0, 0) radius 6 projected
  circle A1 centre (0, 0) radius 5 projected
extrude "Extrusion28" add sketch "Skizze36" against normal blind 6 contours A1
sketch "Skizze37" plane through (0, 0, 30.9) normal (0, 0, 1) x (1, 0, 0)
  circle A0 centre (0, 0) radius 3.5
  dimension "d121" = 7
  constraints: 1 centre point, 1 coincident
  measures "d121" diameter of A0
extrude "Extrusion29" cut sketch "Skizze37" against normal blind 42.5
sketch "Skizze38" plane through (0, 0, 3.8) normal (0, 0, -1) x (-1, 0, 0)
  circle A0 centre (0, 0) radius 31.6258
  constraints: 1 centre point, 1 coincident
extrude "Extrusion30" cut sketch "Skizze38" against normal up to surface (8.1 mm away)
